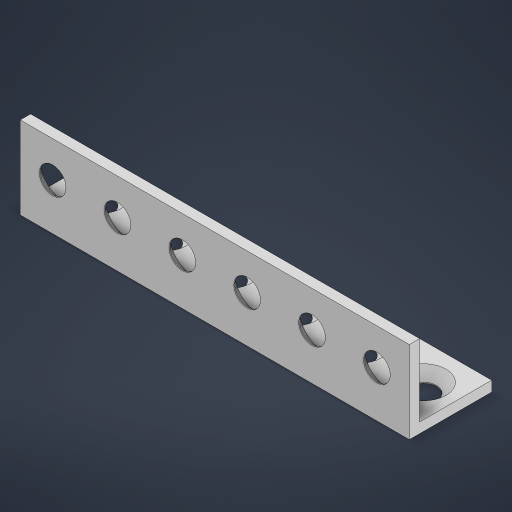
# Autodesk Inventor part: MotorMountingBracket
Saved by Autodesk Inventor 2024 (Build 280153000, 153)
## iProperties
Created: 2024-01-05
Part Number: MotorMountingBracket
Material: Generic
Document SubType Name: Modeling
Designer: avsar
Density: 1 g/cm^3
Appearance: Default
Author: avsar
Autodesk Inventor part; units mm, degrees
ref_plane "YZ Plane" through (0, 0, 0) normal (1, 0, 0) x (0, 1, 0)
ref_plane "XZ Plane" through (0, 0, 0) normal (0, 1, 0) x (-1, 0, 0)
ref_plane "XY Plane" through (0, 0, 0) normal (0, 0, 1) x (1, 0, 0)
sketch "Sketch1" plane through (0, 0, 0) normal (1, 0, 0) x (0, 1, 0)
  line L0 (0, 0) -> (25.4, 0)
  line L1 (0, 0) -> (0, -25.4)
  line L2 (25.4, -3.175) -> (3.175, -3.175)
  line L3 (3.175, -3.175) -> (3.175, -25.4)
  line L4 (3.175, -25.4) -> (0, -25.4)
  line L5 (25.4, 0) -> (25.4, -3.175)
  dimension "d0" = 25.4
  dimension "d1" = 25.4
  dimension "d2" = 3.175
  constraints: 12 end point, 2 horizontal, 2 vertical, 1 other
  measures "d0" distance of L0.start L0.end
  measures "d1" distance of L0.start L1.end
  measures "d2" distance between parallel lines of L0 L2
extrude "Extrusion1" add sketch "Sketch1" along normal mid plane 120
sketch "Sketch2" plane through (-60, 3.175, -3.175) normal (0, 1, 0) x (1, 0, 0)
  circle A0 centre (10, 11.1125) radius 4.1
  line L0 (0, 0) -> (0, 22.225) construction
  line L1 (0, 22.225) -> (120, 22.225) construction
  circle A1 centre (30, 11.1125) radius 4.1
  circle A2 centre (50, 11.1125) radius 4.1
  circle A3 centre (70, 11.1125) radius 4.1
  circle A4 centre (90, 11.1125) radius 4.1
  circle A5 centre (110, 11.1125) radius 4.1
  point P0 (60, -3.175)
  point P1 (0, 11.1125)
  point P2 (0, 11.1125)
  dimension "d5" = 8.2
  dimension "d6" = 10
  dimension "d9" = 20
  constraints: 6 centre point, 2 midpoint, 1 horizontal, 1 horizontal alignment, 10 other
  measures "d5" diameter of A0
  measures "d6" distance of point (0, 11.113) A0.centre
  measures "d9" distance of A0.centre A1.centre
hole "Hole1" at (50, 3.175, -14.2875) at (30, 3.175, -14.2875) at (10, 3.175, -14.2875) at (-10, 3.175, -14.2875) at (-30, 3.175, -14.2875) at (-50, 3.175, -14.2875) direction (0, -1, 0) diameter 8.2 end through all countersink diameter 14 countersink angle 90
sketch "Sketch3" plane through (60, 25.4, -3.175) normal (0, 0, -1) x (-1, 0, 0)
  circle A0 centre (10, -11.1125) radius 4
  line L0 (0, -22.225) -> (0, 0) construction
  line L1 (120, 0) -> (0, 0) construction
  circle A1 centre (30, -11.1125) radius 4
  circle A2 centre (50, -11.1125) radius 4
  circle A3 centre (70, -11.1125) radius 4
  circle A4 centre (90, -11.1125) radius 4
  circle A5 centre (110, -11.1125) radius 4
  point P0 (60, -25.4)
  point P1 (0, -11.1125)
  dimension "d21" = 8
  dimension "d22" = 10
  dimension "d25" = 20
  constraints: 6 centre point, 1 horizontal, 1 horizontal alignment, 1 midpoint, 10 other
  measures "d21" diameter of A0
  measures "d22" distance from line of L0 A0.centre
  measures "d25" distance of A0.centre A1.centre
hole "Hole2" at (50, 14.2875, -3.175) at (30, 14.2875, -3.175) at (10, 14.2875, -3.175) at (-10, 14.2875, -3.175) at (-30, 14.2875, -3.175) at (-50, 14.2875, -3.175) direction (0, 0, 1) diameter 8.2 end through all countersink diameter 14 countersink angle 90
body "Solid1"
